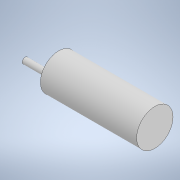
# Autodesk Inventor part: Moteur
Saved by Autodesk Inventor 2020.1 (Build 241239000, 239)
## iProperties
Created: 2019-11-14
Part Number: Moteur
Material: Generic
Document SubType Name: Modeling
Designer: Admin
Density: 1 g/cm^3
Appearance: Default
Author: Admin
Autodesk Inventor part; units mm, degrees
ref_plane "YZ Plane" through (0, 0, 0) normal (1, 0, 0) x (0, 1, 0)
ref_plane "XZ Plane" through (0, 0, 0) normal (0, 1, 0) x (-1, 0, 0)
ref_plane "XY Plane" through (0, 0, 0) normal (0, 0, 1) x (1, 0, 0)
sketch "Sketch1" plane through (0, 0, 0) normal (0, 0, 1) x (1, 0, 0)
  line L0 (-46.4617, 18.5) -> (51.3383, 18.5)
  line L1 (51.3383, 18.5) -> (51.3383, 0)
  line L2 (-46.4617, 18.5) -> (-46.4617, 0)
  line L3 (-46.4617, 0) -> (51.3383, 0)
  point P0 (0, 0)
  dimension "d30" = 97.8
  constraints: 8 end point, 2 vertical, 1 perpendicular
  measures "d30" distance of L0.start L0.end
revolve "Revolution1" add sketch "Sketch1" angle 360 about axis through (-46.4617, 0, 0) along (1, 0, 0)
sketch "Sketch4" plane through (-46.4617, 0, 0) normal (-1, 0, 0) x (0, 0, 1)
  circle A0 centre (0, -7) radius 6
  point P0 (0, 0)
  dimension "d31" = 7
  dimension "d32" = 12
  constraints: 1 centre point
  measures "d31" distance of point (0, 0) A0.centre
  measures "d32" diameter of A0
extrude "Extrusion3" add sketch "Sketch4" along normal blind 7
sketch "Sketch5" plane through (-53.4617, -7, 0) normal (-1, 0, 0) x (0, 0, 1)
  circle A0 centre (0, 0) radius 3
  point P0 (0, 7)
  dimension "d35" = 6
  constraints: 1 centre point
  measures "d35" diameter of A0
extrude "Extrusion4" add sketch "Sketch5" along normal blind 27
body "Solid1"
